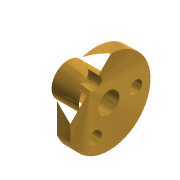
# Autodesk Inventor part: Nut
Saved by Autodesk Inventor 2016 (Build 200138000, 138)
## iProperties
Created: 2016-12-23
Part Number: Nut
Material: Generic
Document SubType Name: Modeling
Designer: inorn
Density: 1 g/cm^3
Appearance: Brass - Satin
Author: inorn
Autodesk Inventor part; units mm, degrees
ref_plane "YZ Plane" through (0, 0, 0) normal (1, 0, 0) x (0, 1, 0)
ref_plane "XZ Plane" through (0, 0, 0) normal (0, 1, 0) x (-1, 0, 0)
ref_plane "XY Plane" through (0, 0, 0) normal (0, 0, 1) x (1, 0, 0)
sketch "Sketch1" plane through (0, 0, 0) normal (1, 0, 0) x (0, 1, 0)
  circle A0 centre (0, 0) radius 4
  dimension "d0" = 8
  constraints: 1 centre point, 1 coincident
  measures "d0" diameter of A0
extrude "Extrusion1" add sketch "Sketch1" along normal blind 9.8
sketch "Sketch2" plane through (9.8, 0, 0) normal (1, 0, 0) x (0, 0, -1)
  circle A0 centre (0, 0) radius 10
  circle A1 centre (0, 0) radius 6.5 construction
  circle A2 centre (0, 6.5) radius 1.5
  circle A3 centre (-5.6292, -3.25) radius 1.5
  circle A4 centre (5.6292, -3.25) radius 1.5
  dimension "d4" = 13
  dimension "d3" = 20
  dimension "d5" = 3
  dimension "d8" = 360
  constraints: 4 centre point, 2 coincident, 1 vertical alignment, 9 other
  measures "d3" diameter of A0
  measures "d5" diameter of A2
extrude "Extrusion2" add sketch "Sketch2" against normal blind 3.2
sketch "Sketch3" plane through (9.8, 0, 0) normal (1, 0, 0) x (0, 0, -1)
  circle A0 centre (0, 0) radius 2.5
  dimension "d12" = 5
  constraints: 1 centre point, 1 coincident
  measures "d12" diameter of A0
extrude "Extrusion3" cut sketch "Sketch3" against normal through all
sketch "Sketch4" plane through (9.8, 0, 0) normal (1, 0, 0) x (0, 0, -1)
  line L0 (8.1454, -10.691) -> (-8.1454, -10.691)
  line L1 (-8.1454, -10.691) -> (-8.1454, -9.309)
  line L2 (-8.1454, -9.309) -> (8.1454, -9.309)
  line L3 (8.1454, -9.309) -> (8.1454, -10.691)
  circle A0 centre (0, 0) radius 10 projected
  line L4 (8.1454, -10.691) -> (-8.1454, -9.309) construction
  line L5 (-8.1454, -10.691) -> (8.1454, -9.309) construction
  point P0 (0, -10)
  constraints: 12 end point, 2 midpoint, 2 parallel, 1 horizontal, 1 perpendicular, 1 vertical alignment, 1 other
extrude "Extrusion4" cut sketch "Sketch4" against normal through all contours L0 L1 L2 A0 L3 | A0 L2 picked at (-0.4144, -9.5135)
body "Solid1"
